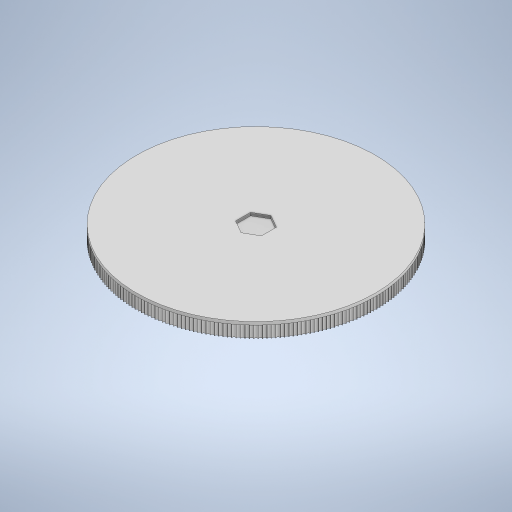
# Autodesk Inventor part: InstrumentalBaraban
Saved by Autodesk Inventor 2024 (Build 280153000, 153)
## iProperties
Created: 2023-08-28
Part Number: InstrumentalBaraban
Material: Generic
Document SubType Name: Modeling
Designer: KirikDK
Density: 1 g/cm^3
Appearance: Default
Author: KirikDK
Autodesk Inventor part; units mm, degrees
ref_plane "YZ Plane" through (0, 0, 0) normal (1, 0, 0) x (0, 1, 0)
ref_plane "XZ Plane" through (0, 0, 0) normal (0, 1, 0) x (-1, 0, 0)
ref_plane "XY Plane" through (0, 0, 0) normal (0, 0, 1) x (1, 0, 0)
sketch "Sketch1" plane through (0, 0, 0) normal (0, 1, 0) x (-1, 0, 0)
  circle A0 centre (0, 0) radius 10
  dimension "d0" = 20
  constraints: 1 centre point, 1 coincident
  measures "d0" diameter of A0
extrude "Extrusion1" add sketch "Sketch1" along normal blind 25
sketch "Sketch2" plane through (0, 25, 0) normal (0, 1, 0) x (1, 0, 0)
  circle A0 centre (0, 0) radius 20
  circle A1 centre (0, 0) radius 10 projected
  dimension "d3" = 40
  constraints: 2 coincident, 1 centre point
  measures "d3" diameter of A0
extrude "Extrusion2" add sketch "Sketch2" along normal blind 2 contours A0 | A1
sketch "Sketch3" plane through (0, 27, 0) normal (0, 1, 0) x (1, 0, 0)
  circle A0 centre (0, 0) radius 80
  dimension "d8" = 160
  constraints: 1 centre point, 1 coincident
  measures "d8" diameter of A0
extrude "Extrusion3" add sketch "Sketch3" along normal blind 10
sketch "Sketch4" plane through (0, 27, 0) normal (0, -1, 0) x (1, 0, 0)
  circle A0 centre (80, 0) radius 1
  point P0 (0, 0)
  constraints: 1 centre point
extrude "Extrusion4" cut sketch "Sketch4" against normal blind 8
pattern_circular "Circular Pattern1" count 240 over 360 about axis through (0, 0, 0) along (0, 1, 0) of "Extrusion4"
sketch "Sketch6" plane through (0, 37, 0) normal (0, 1, 0) x (1, 0, 0)
  line L0 (0, 10) -> (8.6603, 5)
  line L1 (8.6603, 5) -> (8.6603, -5)
  line L2 (8.6603, -5) -> (0, -10)
  line L3 (0, -10) -> (-8.6603, -5)
  line L4 (-8.6603, -5) -> (-8.6603, 5)
  line L5 (-8.6603, 5) -> (0, 10)
  point P0 (0, 0)
  point P1 (0, 0)
  dimension "d17" = 10
  constraints: 12 end point, 1 coincident, 13 other
  measures "d17" distance of L0.start point (0, 0)
extrude "Extrusion5" cut sketch "Sketch6" against normal blind 2
body "Solid1"
